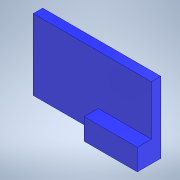
# Autodesk Inventor part: Arduinonano+α
Saved by Autodesk Inventor 2020.2 (Build 242310000, 310)
## iProperties
Created: 2020-03-30
Part Number: Arduinonano+α
Material: 一般
Document SubType Name: Modeling
Designer: aoyama
Mass: 40 g
Surface Area: 160.72 cm^2
Volume: 57.72 cm^3
Density: 0.693001 g/cm^3
Appearance: 青 - 壁塗料 - 光沢
Author: aoyama
Autodesk Inventor part; units mm, degrees
ref_plane "YZ Plane" through (0, 0, 0) normal (1, 0, 0) x (0, 1, 0)
ref_plane "XZ Plane" through (0, 0, 0) normal (0, 1, 0) x (-1, 0, 0)
ref_plane "XY Plane" through (0, 0, 0) normal (0, 0, 1) x (1, 0, 0)
sketch "スケッチ1" plane through (0, 0, 0) normal (0, 0, 1) x (1, 0, 0)
  line L0 (0, 0) -> (-100, 0)
  line L1 (-100, 0) -> (-100, 60)
  line L2 (-100, 60) -> (0, 60)
  line L3 (0, 60) -> (0, 0)
  line L4 (0, 0) -> (-45, 0)
  line L5 (-45, 0) -> (-45, 18)
  line L6 (-45, 18) -> (0, 18)
  line L7 (0, 18) -> (0, 0)
  dimension "d0" = 100
  dimension "d1" = 60
  dimension "d2" = 45
  dimension "d3" = 18
  constraints: 16 end point, 4 parallel, 1 horizontal, 1 vertical
  measures "d0" distance of L1.end L2.end
  measures "d1" distance of L2.end L0.start
  measures "d2" distance of L5.end L6.end
  measures "d3" distance of L4.end L5.end
extrude "押し出し1" add sketch "スケッチ1" along normal blind 8 contours L0 L1 L2 L3 L6 L5
extrude "押し出し2" add sketch "スケッチ1" along normal blind 20 contours L0 L5 L6 L3
